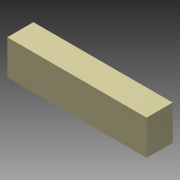
# Autodesk Inventor part: Color sensor
Saved by Autodesk Inventor 2015 (Build 190159000, 159)
## iProperties
Created: 2015-05-26
Part Number: Color sensor
Material: 一般
Document SubType Name: Modeling
Designer: kenta
Density: 1 g/cm^3
Appearance: 既定
Author: kenta
Autodesk Inventor part; units mm, degrees
ref_plane "YZ Plane" through (0, 0, 0) normal (1, 0, 0) x (0, 1, 0)
ref_plane "XZ Plane" through (0, 0, 0) normal (0, 1, 0) x (-1, 0, 0)
ref_plane "XY Plane" through (0, 0, 0) normal (0, 0, 1) x (1, 0, 0)
sketch "スケッチ1" plane through (0, 0, 0) normal (0, 0, 1) x (1, 0, 0)
  line L0 (40, 7.5) -> (-40, 7.5)
  line L1 (-40, 7.5) -> (-40, -7.5)
  line L2 (-40, -7.5) -> (40, -7.5)
  line L3 (40, -7.5) -> (40, 7.5)
  line L4 (40, 7.5) -> (-40, -7.5) construction
  line L5 (-40, 7.5) -> (40, -7.5) construction
  point P0 (0, 0)
  dimension "d0" = 80
  dimension "d1" = 15
  constraints: 12 end point, 2 midpoint, 2 parallel, 1 horizontal, 1 perpendicular
  measures "d0" distance of L2.end L1.end
  measures "d1" distance of L1.end L0.end
extrude "押し出し1" add sketch "スケッチ1" along normal blind 20
